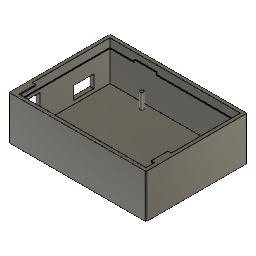
boîte arduino version finale (Autodesk Fusion 360 design; units mm, degrees)
Autodesk Fusion 360 part; units mm, degrees
sketch "Esquisse1" plane through (0, 0, 0) normal (0, 0, 1) x (1, 0, 0)
  line L0 (-37.7016, 28.5178) -> (39.7984, 28.5178)
  line L1 (39.7984, 28.5178) -> (39.7984, -27.4822)
  line L2 (39.7984, -27.4822) -> (-37.7016, -27.4822)
  line L3 (-37.7016, -27.4822) -> (-37.7016, 28.5178)
  dimension "d1" = 77.5
  dimension "d2" = 56
  constraint horizontal L0
  constraint vertical L1
  constraint horizontal L2
  constraint vertical L3
  measures "d1" distance of L0.start L0.end
  measures "d2" distance of L0 L2
extrude "Extrusion1" add sketch "Esquisse1" along normal blind 19
sketch "Esquisse2" plane through (0, 0, 19) normal (0, 0, 1) x (-1, 0, 0)
  line L0 (37.7016, 27.4822) -> (-39.7984, 27.4822)
  line L1 (-39.7984, 27.4822) -> (-39.7984, -28.5178)
  line L2 (-39.7984, -28.5178) -> (37.7016, -28.5178)
  line L3 (37.7016, -28.5178) -> (37.7016, 27.4822)
  line L4 (-39.2984, -28.0178) -> (37.2016, -28.0178)
  line L5 (37.2016, -28.0178) -> (37.2016, 26.9822)
  line L6 (37.2016, 26.9822) -> (-39.2984, 26.9822)
  line L7 (-39.2984, 26.9822) -> (-39.2984, -28.0178)
  dimension "d5" = -0.5
extrude "Extrusion2" cut sketch "Esquisse2" against normal blind 15 contours L4 L5 L6 L7
sketch "Esquisse5" plane through (0, 0, 4) normal (0, 0, 1) x (-1, 0, 0)
  line L0 (-39.2984, 26.9822) -> (-39.2984, -28.0178)
  line L1 (-39.2984, -28.0178) -> (37.2016, -28.0178)
  line L2 (37.2016, -28.0178) -> (37.2016, 26.9822)
  line L3 (37.2016, 26.9822) -> (-39.2984, 26.9822)
  line L4 (37.7016, 27.4822) -> (-39.7984, 27.4822)
  line L5 (-39.2984, 26.9822) -> (37.2016, 26.9822)
  line L6 (37.2016, -28.0178) -> (-39.2984, -28.0178)
  line L7 (-39.7984, -28.5178) -> (37.7016, -28.5178)
  line L8 (-24.7984, 27.4822) -> (-11.7984, 27.4822)
  line L9 (-11.7984, 27.4822) -> (-11.7984, 26.9822)
  line L10 (-11.7984, 26.9822) -> (-24.7984, 26.9822)
  line L11 (-24.7984, 26.9822) -> (-24.7984, 27.4822)
  line L12 (9.7016, -28.0178) -> (22.7016, -28.0178)
  line L13 (22.7016, -28.0178) -> (22.7016, -28.5178)
  line L14 (22.7016, -28.5178) -> (9.7016, -28.5178)
  line L15 (9.7016, -28.5178) -> (9.7016, -28.0178)
  line L16 (-39.7984, 27.4822) -> (-39.7984, -28.5178)
  line L17 (-39.2984, -28.0178) -> (-39.2984, 26.9822)
  line L18 (37.2016, 26.9822) -> (37.2016, -28.0178)
  line L19 (37.7016, -28.5178) -> (37.7016, 27.4822)
  dimension "d11" = 13
  dimension "d12" = 13
  dimension "d13" = 15
  dimension "d14" = 15
  constraint horizontal L8
  constraint vertical L9
  constraint horizontal L10
  constraint vertical L11
  constraint coincident L4 L8.start
  constraint horizontal L12
  constraint vertical L13
  constraint horizontal L14
  constraint vertical L15
  constraint coincident L6 L12.start
  measures "d11" distance of L8.start L8.end
  measures "d12" distance of L12.start L12.end
  measures "d13" distance of L11 L16
  measures "d14" distance of L13 L19
extrude "Extrusion3" add sketch "Esquisse5" along normal blind 16.5 contours L3 L4 L5 L8 L9 L10 L11 | L1 L6 L7 L12 L13 L14 L15
sketch "Esquisse6" plane through (0, 0, 4) normal (0, 0, 1) x (-1, 0, 0)
  line L0 (-39.2984, 26.9822) -> (-39.2984, -28.0178)
  line L1 (-39.2984, -28.0178) -> (37.2016, -28.0178)
  line L2 (37.2016, -28.0178) -> (37.2016, 26.9822)
  line L3 (37.2016, 26.9822) -> (-39.2984, 26.9822)
  circle A0 centre (14.7016, -24.5178) radius 1
  circle A1 centre (17.2016, 23.4822) radius 1
  line L4 (37.7016, -28.5178) -> (37.7016, 27.4822)
  line L5 (9.7016, -28.5178) -> (22.7016, -28.5178)
  line L6 (37.7016, 27.4822) -> (-11.7984, 27.4822)
  dimension "d17" = 2
  dimension "d18" = 2
  dimension "d22" = 4
  dimension "d23" = 4
  dimension "d49" = 20
  dimension "d50" = 22.5
  measures "d17" diameter of A0
  measures "d18" diameter of A1
  measures "d22" distance of A0.centre L5
  measures "d23" distance of A1.centre L6
  measures "d49" distance of L2 A1.centre
  measures "d50" distance of L2 A0.centre
extrude "Extrusion4" add sketch "Esquisse6" along normal blind 6 contours A0 | A1
sketch "Esquisse7" plane through (-37.7016, 0, 0) normal (-1, 0, 0) x (0, -1, 0)
  line L0 (-28.5178, 0) -> (27.4822, 0)
  line L1 (27.4822, 0) -> (27.4822, 19)
  line L2 (27.4822, 19) -> (-28.5178, 19)
  line L3 (-28.5178, 19) -> (-28.5178, 0)
  line L4 (-18.5178, 10.6) -> (-6.5178, 10.6)
  line L5 (-6.5178, 10.6) -> (-6.5178, 3.1)
  line L6 (-6.5178, 3.1) -> (-18.5178, 3.1)
  line L7 (-18.5178, 3.1) -> (-18.5178, 10.6)
  line L8 (13.4822, 17.1) -> (21.9822, 17.1)
  line L9 (21.9822, 17.1) -> (21.9822, 4.1)
  line L10 (21.9822, 4.1) -> (13.4822, 4.1)
  line L11 (13.4822, 4.1) -> (13.4822, 17.1)
  dimension "d26" = 12
  dimension "d27" = 7.5
  dimension "d28" = 10
  dimension "d29" = 8.5
  dimension "d30" = 13
  dimension "d31" = 5.5
  dimension "d32" = 4.1
  dimension "d33" = 3.1
  constraint horizontal L4
  constraint vertical L5
  constraint horizontal L6
  constraint vertical L7
  constraint horizontal L8
  constraint vertical L9
  constraint horizontal L10
  constraint vertical L11
  measures "d26" distance of L4.start L4.end
  measures "d27" distance of L4 L6
  measures "d28" distance of L3 L7
  measures "d29" distance of L8.start L8.end
  measures "d30" distance of L8.start L10.end
  measures "d31" distance of L1 L9
  measures "d32" distance of L0 L10
  measures "d33" distance of L0 L6
extrude "Extrusion5" cut sketch "Esquisse7" against normal blind 33 contours L4 L5 L6 L7 | L8 L9 L10 L11
extrude "Extrusion6" cut sketch "Esquisse6" against normal blind 3
extrude "Extrusion7" add 1 faces at (-11.8683, 9.8511, 0) along direction (0, 0, -1) blind 2
sketch "Esquisse8" plane through (0, 0, 0) normal (0, 0, 1) x (1, 0, 0)
  line L0 (39.7984, 28.5178) -> (-9.7016, 28.5178)
  line L1 (-9.7016, 28.5178) -> (-22.7016, 28.5178)
  line L2 (-22.7016, 28.5178) -> (-37.7016, 28.5178)
  line L3 (-37.7016, 28.5178) -> (-37.7016, -27.4822)
  line L4 (39.7984, -27.4822) -> (39.7984, 28.5178)
  line L5 (24.7984, -27.4822) -> (39.7984, -27.4822)
  line L6 (11.7984, -27.4822) -> (24.7984, -27.4822)
  line L7 (-37.7016, -27.4822) -> (11.7984, -27.4822)
  line L8 (24.7984, -29.4822) -> (41.7984, -29.4822)
  line L9 (41.7984, -29.4822) -> (41.7984, 30.5178)
  line L10 (41.7984, 30.5178) -> (-9.7016, 30.5178)
  line L11 (-9.7016, 30.5178) -> (-22.7016, 30.5178)
  line L12 (-22.7016, 30.5178) -> (-39.7016, 30.5178)
  line L13 (-39.7016, 30.5178) -> (-39.7016, -29.4822)
  line L14 (-39.7016, -29.4822) -> (11.7984, -29.4822)
  line L15 (11.7984, -29.4822) -> (24.7984, -29.4822)
  dimension "d40" = 2
extrude "Extrusion8" add sketch "Esquisse8" along normal blind 24 and the other way blind 2
extrude "Extrusion9" cut 2 faces at (-37.7016, -16.3155, 8.4333) (-37.7016, 14.5178, 5.6) along direction (1, 0, 0) blind 0 and the other way blind 5
extrude "Extrusion10" add sketch "Esquisse6" along normal blind 6 and the other way blind 2 contours A1
sketch "Esquisse9" plane through (39.7984, 0, 0) normal (-1, 0, 0) x (0, -1, 0)
  line L0 (-28.5178, 19) -> (27.4822, 19)
  line L1 (27.4822, 19) -> (27.4822, 24)
  line L2 (27.4822, 24) -> (-28.5178, 24)
  line L3 (-28.5178, 24) -> (-28.5178, 19)
  line L4 (12.4822, 24) -> (22.4822, 24)
  line L5 (22.4822, 24) -> (22.4822, 23.3)
  line L6 (22.4822, 23.3) -> (12.4822, 23.3)
  line L7 (12.4822, 23.3) -> (12.4822, 24)
  dimension "d55" = 10
  dimension "d56" = 0.7
  dimension "d57" = 5
  constraint horizontal L4
  constraint vertical L5
  constraint horizontal L6
  constraint vertical L7
  constraint coincident L2 L4.start
  measures "d55" distance of L4.start L4.end
  measures "d56" distance of L4.start L6.end
  measures "d57" distance of L1 L5
extrude "Extrusion11" add sketch "Esquisse9" along normal blind 2 contours L2 L4 L5 L6 L7
sketch "Esquisse10" plane through (-37.7016, 0, 0) normal (1, 0, 0) x (0, 1, 0)
  line L0 (-27.4822, 19) -> (28.5178, 19)
  line L1 (28.5178, 19) -> (28.5178, 24)
  line L2 (28.5178, 24) -> (-27.4822, 24)
  line L3 (-27.4822, 24) -> (-27.4822, 19)
  line L4 (-27.4822, 24) -> (-17.4822, 24)
  line L5 (-17.4822, 24) -> (-17.4822, 23.3)
  line L6 (-17.4822, 23.3) -> (-27.4822, 23.3)
  line L7 (-27.4822, 23.3) -> (-27.4822, 24)
  dimension "d60" = 10
  dimension "d61" = 0.7
  constraint horizontal L4
  constraint vertical L5
  constraint horizontal L6
  constraint vertical L7
  constraint coincident L2 L3.start
  constraint coincident L3 L2.end
  measures "d60" distance of L2.end L4.end
  measures "d61" distance of L2.end L6.end
extrude "Extrusion12" add sketch "Esquisse10" along normal blind 2 contours L2 L3 L4 L5 L6 L7
fillet "Congé1" radius 0.45 4 edges at (41.7984, -29.4822, 11) (41.7984, 30.5178, 11) (-39.7016, 30.5178, 11) (-39.7016, -29.4822, 11)
equation "d1 = LongueurBoite"
equation "d2 = LargeurBoite"
equation "d26 = LargeurTrouUSB"
equation "d27 = HauteurTrouUSB"
equation "d28 = DistanceBordTrouUSB"
equation "d29 = LargeurTrouAC"
equation "d30 = HauteurTrouAC"
equation "d31 = DistanceBordTrouAC"
equation "d32 = DistanceDessousTrouAC"
equation "d33 = DistanceDessousTrouUSB"
equation "LargeurBoite = 56 mm"
equation "LongueurBoite = 77.5 mm"
equation "LargeurTrouAC = 8.5 mm"
equation "HauteurTrouAC = 13 mm"
equation "LargeurTrouUSB = 12 mm"
equation "HauteurTrouUSB = 7.5 mm"
equation "DistanceBordTrouUSB = 10 mm"
equation "DistanceBordTrouAC = 5.5 mm"
equation "DistanceDessousTrouUSB = 3.1 mm"
equation "DistanceDessousTrouAC = 4.1 mm"
